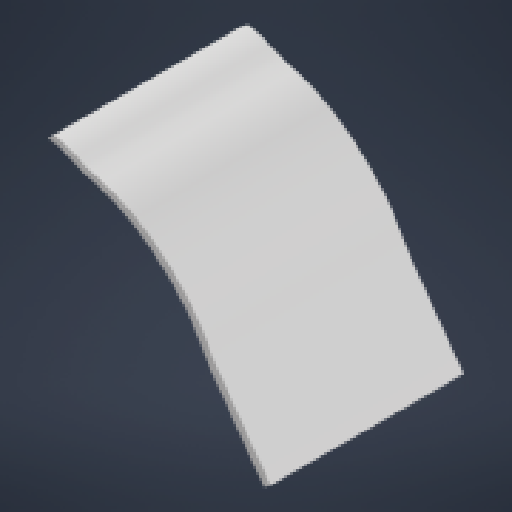
# Autodesk Inventor part: intake
Saved by Autodesk Inventor 2023.2 (Build 272271000, 271)
## iProperties
Created: 2023-03-29
Part Number: intake
Material: Generic
Document SubType Name: Modeling
Designer: Liam
Density: 1 g/cm^3
Appearance: Default
Author: Liam
Autodesk Inventor part; units mm, degrees
ref_plane "YZ Plane" through (0, 0, 0) normal (1, 0, 0) x (0, 1, 0)
ref_plane "XZ Plane" through (0, 0, 0) normal (0, 1, 0) x (-1, 0, 0)
ref_plane "XY Plane" through (0, 0, 0) normal (0, 0, 1) x (1, 0, 0)
sketch "Sketch1" plane through (0, 0, 0) normal (0, 0, 1) x (1, 0, 0)
  line L0 (-43.4306, 216.1135) -> (-31.9999, 213.9599) construction
  line L1 (-31.9999, 213.9599) -> (-25.0421, 208.493) construction
  line L2 (-25.0421, 208.493) -> (-10.6294, 205.8424) construction
  line L3 (-10.6294, 205.8424) -> (3.6175, 200.0442) construction
  line L4 (3.6175, 200.0442) -> (22.6687, 189.2762) construction
  line L5 (22.6687, 189.2762) -> (43.3764, 169.2311) construction
  line L6 (43.3764, 169.2311) -> (52.9849, 156.4751) construction
  line L7 (52.9849, 156.4751) -> (60.4397, 141.5655) construction
  line L8 (60.4397, 141.5655) -> (62.5933, 138.7492) construction
  line L9 (62.5933, 138.7492) -> (76.6746, 118.3728) construction
  line L10 (76.6746, 118.3728) -> (98.542, 88.0566) construction
  spline S0 degree 4 poles (-43.4306, 216.1135) (-31.9999, 213.9599) (-25.0421, 208.493) (-10.6294, 205.8424) (3.6175, 200.0442) (22.6687, 189.2762) (43.3764, 169.2311) (52.9849, 156.4751) (60.4397, 141.5655) (62.5933, 138.7492) (76.6746, 118.3728) (98.542, 88.0566) knots 1 1 1 1 1 2 3 4 5 6 7 8 9 9 9 9 9
  line L11 (-47.5934, 212.7512) -> (-36.1627, 210.5976) construction
  line L12 (-36.1627, 210.5976) -> (-29.2049, 205.1308) construction
  line L13 (-29.2049, 205.1308) -> (-14.7923, 202.4802) construction
  line L14 (-14.7923, 202.4802) -> (-0.5453, 196.682) construction
  line L15 (-0.5453, 196.682) -> (18.5058, 185.914) construction
  line L16 (18.5058, 185.914) -> (39.2136, 165.8688) construction
  line L17 (39.2136, 165.8688) -> (48.822, 153.1128) construction
  line L18 (48.822, 153.1128) -> (56.2768, 138.2032) construction
  line L19 (56.2768, 138.2032) -> (58.4304, 135.387) construction
  line L20 (58.4304, 135.387) -> (72.5117, 115.0105) construction
  line L21 (72.5117, 115.0105) -> (94.3791, 84.6943) construction
  spline S1 degree 4 poles (-47.5934, 212.7512) (-36.1627, 210.5976) (-29.2049, 205.1308) (-14.7923, 202.4802) (-0.5453, 196.682) (18.5058, 185.914) (39.2136, 165.8688) (48.822, 153.1128) (56.2768, 138.2032) (58.4304, 135.387) (72.5117, 115.0105) (94.3791, 84.6943) knots 1 1 1 1 1 2 3 4 5 6 7 8 9 9 9 9 9
  line L22 (94.3791, 84.6943) -> (98.542, 88.0566)
  line L23 (-47.5934, 212.7512) -> (-43.4306, 216.1135)
  point P0 (0, 0)
  constraints: 4 end point, 1 parallel, 6 other
extrude "Extrusion1" add sketch "Sketch1" along normal blind 127
body "Solid1"
